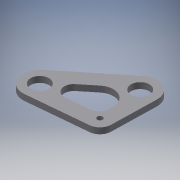
# Autodesk Inventor part: tipper_link_B
Saved by Autodesk Inventor 2017.2 (Build 212233000, 233)
## iProperties
Created: 2017-07-15
Part Number: tipper_link_B
Material: Generic
Document SubType Name: Modeling
Designer: Nic
Density: 1 g/cm^3
Appearance: Default
Author: Nic
Autodesk Inventor part; units mm, degrees
ref_plane "YZ Plane" through (0, 0, 0) normal (1, 0, 0) x (0, 1, 0)
ref_plane "XZ Plane" through (0, 0, 0) normal (0, 1, 0) x (-1, 0, 0)
ref_plane "XY Plane" through (0, 0, 0) normal (0, 0, 1) x (1, 0, 0)
sketch "Sketch1" plane through (0, 0, 0) normal (0, 0, 1) x (1, 0, 0)
  circle A0 centre (0, 0) radius 1.45
  arc A1 (-37.6548, 7.0016) -> (-31.1562, -8.9604) centre (-32, 0) ccw
  line L0 (-31.1562, -8.9604) -> (0.5625, -5.9736)
  circle A2 centre (-32, 0) radius 4.85
  line L1 (0, 0) -> (-32, 0) construction
  arc A3 (0.5625, -5.9736) -> (5.9983, -0.1415) centre (0, 0) ccw
  circle A4 centre (-2.4375, 23.8759) radius 4.85
  arc A5 (6.56, 23.6636) -> (-8.0923, 30.8775) centre (-2.4375, 23.8759) ccw
  line L2 (-37.6548, 7.0016) -> (-8.0923, 30.8775)
  line L3 (6.56, 23.6636) -> (5.9983, -0.1415)
  line L4 (-14.8184, 15.162) -> (-22.3039, 9.1163)
  line L5 (-18.6936, 0.2486) -> (-6.3825, 1.4078)
  line L6 (-1.8527, 6.2679) -> (-1.7941, 8.7496)
  arc A6 (-22.3039, 9.1163) -> (-18.6936, 0.2486) centre (-19.1624, 5.2265) ccw
  arc A7 (-1.7941, 8.7496) -> (-14.8184, 15.162) centre (-9.7919, 8.9383) ccw
  arc A8 (-6.3825, 1.4078) -> (-1.8527, 6.2679) centre (-6.8513, 6.3858) ccw
  dimension "d0" = 2.9
  dimension "d2" = 32
  dimension "d61" = 6
  dimension "d62" = 38
  dimension "d63" = 24
  dimension "d64" = 8
  dimension "d66" = 8
  dimension "d67" = 5
  dimension "d68" = 9.7
  dimension "d69" = 9
  dimension "d70" = 9.7
  dimension "d71" = 5
  constraints: 14 end point, 12 point on circle, 12 tangent, 9 centre point, 3 coincident, 1 concentric, 1 equal radius, 1 horizontal, 1 point on line, 2 other
  measures "d0" diameter of A0
  measures "d2" distance of point (0, 0) A1.centre
  measures "d61" radius of A3
  measures "d62" distance of A4.centre A1.centre
  measures "d63" distance of point (0, 0) A4.centre
  measures "d64" distance between parallel lines of L2 L4
  measures "d66" radius of A7
  measures "d67" radius of A8
  measures "d68" diameter of A4
  measures "d69" radius of A5
  measures "d70" diameter of A2
  measures "d71" radius of A6
extrude "Extrusion1" add sketch "Sketch1" along normal blind 3.175
body "Solid1"
